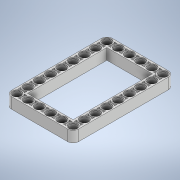
# Autodesk Inventor part: vehicle-adapter
Saved by Autodesk Inventor 2021 (Build 250183000, 183)
## iProperties
Created: 2024-03-15
Part Number: vehicle-adapter
Material: Generic
Document SubType Name: Modeling
Designer: 22hamfri
Density: 1 g/cm^3
Appearance: Default
Author: 22hamfri
Autodesk Inventor part; units mm, degrees
ref_plane "YZ Plane" through (0, 0, 0) normal (1, 0, 0) x (0, 1, 0)
ref_plane "XZ Plane" through (0, 0, 0) normal (0, 1, 0) x (-1, 0, 0)
ref_plane "XY Plane" through (0, 0, 0) normal (0, 0, 1) x (1, 0, 0)
sketch "Sketch1" plane through (0, 0, 0) normal (0, 1, 0) x (-1, 0, 0)
  line L0 (-16.125, 28.08) -> (16.125, 28.08)
  line L1 (16.125, 28.08) -> (16.125, -28.08)
  line L2 (16.125, -28.08) -> (-16.125, -28.08)
  line L3 (-16.125, -28.08) -> (-16.125, 28.08)
  line L4 (-16.125, 28.08) -> (16.125, -28.08) construction
  line L5 (16.125, 28.08) -> (-16.125, -28.08) construction
  circle A0 centre (3.985, -31.88) radius 2.575
  circle A1 centre (3.985, -31.88) radius 3.1
  circle A2 centre (3.985, -31.88) radius 3.8
  circle A3 centre (11.955, -31.88) radius 2.575
  circle A4 centre (11.955, -31.88) radius 3.1
  circle A5 centre (11.955, -31.88) radius 3.8
  circle A6 centre (19.925, -31.88) radius 2.575
  circle A7 centre (19.925, -31.88) radius 3.1
  circle A8 centre (19.925, -31.88) radius 3.8
  circle A9 centre (19.925, -23.91) radius 2.575
  circle A10 centre (19.925, -23.91) radius 3.1
  circle A11 centre (19.925, -23.91) radius 3.8
  circle A12 centre (19.925, -15.94) radius 2.575
  circle A13 centre (19.925, -15.94) radius 3.1
  circle A14 centre (19.925, -15.94) radius 3.8
  circle A15 centre (19.925, -7.97) radius 2.575
  circle A16 centre (19.925, -7.97) radius 3.1
  circle A17 centre (19.925, -7.97) radius 3.8
  circle A18 centre (19.925, 0) radius 2.575
  circle A19 centre (19.925, 0) radius 3.1
  circle A20 centre (19.925, 0) radius 3.8
  line L6 (-23.725, 35.68) -> (23.725, 35.68)
  line L7 (23.725, 35.68) -> (23.725, -35.68)
  line L8 (23.725, -35.68) -> (-23.725, -35.68)
  line L9 (-23.725, -35.68) -> (-23.725, 35.68)
  line L10 (-23.725, 35.68) -> (23.725, -35.68) construction
  line L11 (23.725, 35.68) -> (-23.725, -35.68) construction
  line L12 (23.725, 0) -> (-23.725, 0)
  line L13 (22.225, -3.0249) -> (22.225, -4.9451)
  line L14 (22.225, -10.9949) -> (22.225, -12.9151)
  line L15 (22.225, -18.9649) -> (22.225, -20.8851)
  line L16 (22.225, -26.9349) -> (22.225, -28.8551)
  line L17 (19.925, 0) -> (19.925, -31.88)
  line L18 (17.625, -3.0249) -> (17.625, -4.9451)
  line L19 (17.625, -10.9949) -> (17.625, -12.9151)
  line L20 (17.625, -18.9649) -> (17.625, -20.8851)
  line L21 (17.625, -26.9349) -> (17.625, -28.8551)
  line L22 (16.9001, -34.18) -> (14.9799, -34.18)
  line L23 (8.9301, -34.18) -> (7.0099, -34.18)
  line L24 (19.925, -31.88) -> (3.985, -31.88)
  line L25 (16.9001, -29.58) -> (14.9799, -29.58)
  line L26 (8.9301, -29.58) -> (7.0099, -29.58)
  line L27 (0, 35.68) -> (0, -35.68)
  line L28 (-16.125, 28.08) -> (-16.125, -28.08)
  line L29 (-16.125, -28.08) -> (16.125, -28.08)
  line L30 (16.125, 28.08) -> (-16.125, -28.08) construction
  line L31 (-16.125, 28.08) -> (16.125, -28.08) construction
  circle A21 centre (-3.985, -31.88) radius 2.575
  circle A22 centre (-3.985, -31.88) radius 3.1
  circle A23 centre (-3.985, -31.88) radius 3.8
  circle A24 centre (-11.955, -31.88) radius 2.575
  circle A25 centre (-11.955, -31.88) radius 3.1
  circle A26 centre (-11.955, -31.88) radius 3.8
  circle A27 centre (-19.925, -31.88) radius 2.575
  circle A28 centre (-19.925, -31.88) radius 3.1
  circle A29 centre (-19.925, -31.88) radius 3.8
  circle A30 centre (-19.925, -23.91) radius 2.575
  circle A31 centre (-19.925, -23.91) radius 3.1
  circle A32 centre (-19.925, -23.91) radius 3.8
  circle A33 centre (-19.925, -15.94) radius 2.575
  circle A34 centre (-19.925, -15.94) radius 3.1
  circle A35 centre (-19.925, -15.94) radius 3.8
  circle A36 centre (-19.925, -7.97) radius 2.575
  circle A37 centre (-19.925, -7.97) radius 3.1
  circle A38 centre (-19.925, -7.97) radius 3.8
  circle A39 centre (-19.925, 0) radius 2.575
  circle A40 centre (-19.925, 0) radius 3.1
  circle A41 centre (-19.925, 0) radius 3.8
  line L32 (-23.725, 35.68) -> (-23.725, -35.68)
  line L33 (-23.725, -35.68) -> (23.725, -35.68)
  line L34 (23.725, 35.68) -> (-23.725, -35.68) construction
  line L35 (-23.725, 35.68) -> (23.725, -35.68) construction
  line L36 (-23.725, 0) -> (23.725, 0)
  line L37 (-22.225, -3.0249) -> (-22.225, -4.9451)
  line L38 (-22.225, -10.9949) -> (-22.225, -12.9151)
  line L39 (-22.225, -18.9649) -> (-22.225, -20.8851)
  line L40 (-22.225, -26.9349) -> (-22.225, -28.8551)
  line L41 (-19.925, 0) -> (-19.925, -31.88)
  line L42 (-17.625, -3.0249) -> (-17.625, -4.9451)
  line L43 (-17.625, -10.9949) -> (-17.625, -12.9151)
  line L44 (-17.625, -18.9649) -> (-17.625, -20.8851)
  line L45 (-17.625, -26.9349) -> (-17.625, -28.8551)
  line L46 (-16.9001, -34.18) -> (-14.9799, -34.18)
  line L47 (-8.9301, -34.18) -> (-7.0099, -34.18)
  line L48 (-19.925, -31.88) -> (-3.985, -31.88)
  line L49 (-16.9001, -29.58) -> (-14.9799, -29.58)
  line L50 (-8.9301, -29.58) -> (-7.0099, -29.58)
  line L51 (0.9601, -34.18) -> (-0.9601, -34.18)
  line L52 (0.9601, -29.58) -> (-0.9601, -29.58)
  line L53 (16.125, 28.08) -> (-16.125, 28.08)
  circle A42 centre (3.985, 31.88) radius 2.575
  circle A43 centre (3.985, 31.88) radius 3.1
  circle A44 centre (3.985, 31.88) radius 3.8
  circle A45 centre (11.955, 31.88) radius 2.575
  circle A46 centre (11.955, 31.88) radius 3.1
  circle A47 centre (11.955, 31.88) radius 3.8
  circle A48 centre (19.925, 31.88) radius 2.575
  circle A49 centre (19.925, 31.88) radius 3.1
  circle A50 centre (19.925, 31.88) radius 3.8
  circle A51 centre (19.925, 23.91) radius 2.575
  circle A52 centre (19.925, 23.91) radius 3.1
  circle A53 centre (19.925, 23.91) radius 3.8
  circle A54 centre (19.925, 15.94) radius 2.575
  circle A55 centre (19.925, 15.94) radius 3.1
  circle A56 centre (19.925, 15.94) radius 3.8
  circle A57 centre (19.925, 7.97) radius 2.575
  circle A58 centre (19.925, 7.97) radius 3.1
  circle A59 centre (19.925, 7.97) radius 3.8
  circle A60 centre (19.925, 0) radius 2.575
  circle A61 centre (19.925, 0) radius 3.1
  circle A62 centre (19.925, 0) radius 3.8
  line L54 (23.725, 35.68) -> (-23.725, 35.68)
  line L55 (22.225, 3.0249) -> (22.225, 4.9451)
  line L56 (22.225, 10.9949) -> (22.225, 12.9151)
  line L57 (22.225, 18.9649) -> (22.225, 20.8851)
  line L58 (22.225, 26.9349) -> (22.225, 28.8551)
  line L59 (19.925, 0) -> (19.925, 31.88)
  line L60 (17.625, 3.0249) -> (17.625, 4.9451)
  line L61 (17.625, 10.9949) -> (17.625, 12.9151)
  line L62 (17.625, 18.9649) -> (17.625, 20.8851)
  line L63 (17.625, 26.9349) -> (17.625, 28.8551)
  line L64 (16.9001, 34.18) -> (14.9799, 34.18)
  line L65 (8.9301, 34.18) -> (7.0099, 34.18)
  line L66 (19.925, 31.88) -> (3.985, 31.88)
  line L67 (16.9001, 29.58) -> (14.9799, 29.58)
  line L68 (8.9301, 29.58) -> (7.0099, 29.58)
  circle A63 centre (-3.985, 31.88) radius 2.575
  circle A64 centre (-19.925, 15.94) radius 3.1
  circle A65 centre (-19.925, 31.88) radius 2.575
  circle A66 centre (-19.925, 0) radius 2.575
  circle A67 centre (-19.925, 0) radius 3.1
  circle A68 centre (-19.925, 0) radius 3.8
  circle A69 centre (-19.925, 7.97) radius 2.575
  circle A70 centre (-19.925, 7.97) radius 3.1
  circle A71 centre (-19.925, 7.97) radius 3.8
  circle A72 centre (-19.925, 15.94) radius 2.575
  circle A73 centre (-19.925, 23.91) radius 2.575
  circle A74 centre (-19.925, 23.91) radius 3.1
  circle A75 centre (-19.925, 23.91) radius 3.8
  circle A76 centre (-11.955, 31.88) radius 3.8
  circle A77 centre (-11.955, 31.88) radius 2.575
  circle A78 centre (-11.955, 31.88) radius 3.1
  circle A79 centre (-3.985, 31.88) radius 3.1
  circle A80 centre (-3.985, 31.88) radius 3.8
  circle A81 centre (-19.925, 31.88) radius 3.1
  circle A82 centre (-19.925, 31.88) radius 3.8
  circle A83 centre (-19.925, 15.94) radius 3.8
  line L69 (-16.125, 28.08) -> (16.125, 28.08)
  line L70 (-17.625, 3.0249) -> (-17.625, 4.9451)
  line L71 (-22.225, 3.0249) -> (-22.225, 4.9451)
  line L72 (-17.625, 10.9949) -> (-17.625, 12.9151)
  line L73 (-22.225, 10.9949) -> (-22.225, 12.9151)
  line L74 (-17.625, 18.9649) -> (-17.625, 20.8851)
  line L75 (-19.925, 0) -> (-19.925, 31.88)
  line L76 (-23.725, 35.68) -> (23.725, 35.68)
  line L77 (-22.225, 26.9349) -> (-22.225, 28.8551)
  line L78 (-22.225, 18.9649) -> (-22.225, 20.8851)
  line L79 (-17.625, 26.9349) -> (-17.625, 28.8551)
  line L80 (-16.9001, 29.58) -> (-14.9799, 29.58)
  line L81 (-8.9301, 29.58) -> (-7.0099, 29.58)
  line L82 (-19.925, 31.88) -> (-3.985, 31.88)
  line L83 (-8.9301, 34.18) -> (-7.0099, 34.18)
  line L84 (-16.9001, 34.18) -> (-14.9799, 34.18)
  line L85 (0.9601, 34.18) -> (-0.9601, 34.18)
  line L86 (0.9601, 29.58) -> (-0.9601, 29.58)
  point P0 (0, 0)
  point P1 (19.925, -35.68)
  point P2 (23.725, -31.88)
  point P3 (23.725, 31.88)
  point P4 (19.925, 35.68)
  point P5 (-19.925, 35.68)
  point P6 (-23.725, 31.88)
  point P7 (-23.725, -31.88)
  point P8 (-19.925, -35.68)
  point P9 (-16.825, 0)
  point P10 (-17.35, 0)
  point P11 (-22.5, 0)
  point P12 (-23.025, 0)
  dimension "d0" = 5.15
  dimension "d1" = 6.2
  dimension "d2" = 0.7
  dimension "d5" = 7.97
  dimension "d12" = 7.97
  dimension "d17" = 1.5
  dimension "d18" = 1.5
  dimension "d19" = 7.97
  dimension "d20" = 1.5
  dimension "d21" = 1.5
  constraints: 174 end point, 125 symmetric about line, 80 centre point, 52 point on circle, 9 parallel, 8 midpoint, 6 horizontal, 5 vertical, 4 collinear, 3 tangent, 2 perpendicular, 2 point on line, 95 other
  measures "d0" diameter of A0
  measures "d1" diameter of A1
  measures "d2" radial gap between concentric circles of A1 A2
  measures "d5" distance of L24.end A3.centre
  measures "d12" distance of L17.end A9.centre
  measures "d17" distance between parallel lines of L7 L14
  measures "d18" distance between parallel lines of L8 L22
  measures "d19" distance of L48.end L24.end
  measures "d20" distance between parallel lines of L33 L51
  measures "d21" distance between parallel lines of L2 L52
extrude "Extrusion1" add sketch "Sketch1" against normal mid plane 7.76 contours L3 A75 L79 A82 L80 A76 L0 | A76 L81 A80 L0 | A76 L82 A78 | A75 L75 A74 | L3 A83 L74 A75 | A80 L86 L27 L0 | A80 | A83 L75 A64 | L3 A71 L72 A83 | L27 L86 A44 L0 | A76 L82 A78 | A82 L75 A81 L82 | A71 L75 A70 | L3 A41 L70 A71 | L75 A74 A75 | A44 L68 A47 L0 | A44 | L84 A82 L6 A76 | L82 A81 L75 A82 | A76 L6 A80 L83 | A41 L41 A40 L12 | L12 A40 L75 A41 | L3 A38 L42 A41 | L75 A64 A83 | A75 L9 A82 L77 | L78 A83 L9 A75 | A47 L67 A50 L63 A53 L1 L0 | A47 L66 A46 | L85 A80 L6 L27 | L27 L6 A44 L85 | A20 L18 A17 L1 | L1 A59 L60 A20 | L12 A19 L17 A20 | A20 L59 A19 L12 | L27 L52 A23 L2 | L2 A2 L52 L27 | A38 L41 A37 | L3 A35 L43 A38 | L75 A70 A71 | L73 A71 L9 A83 | L1 A56 L61 A59 | A59 L59 A58 | A17 L19 A14 L1 | A17 L17 A16 | L2 A5 L26 A2 | A2 | A23 L50 A26 L2 | A23 | A35 L41 A34 | L3 A32 L44 A35 | A40 L12 A41 L75 | L41 A41 L12 A40 | L71 A41 L9 A71 | A53 L62 A56 L1 | A53 L59 A52 | A47 L66 A46 | A50 L66 A49 L59 | L6 A47 L65 A44 | A56 L59 A55 | A14 L20 A11 L1 | A14 L17 A13 | A20 L12 A19 L59 | L17 A19 L12 A20 | L2 L1 A11 L21 A8 L25 A5 | A5 L24 A4 | A26 L49 A29 L45 A32 L3 L2 | A26 L48 A25 | L51 A2 L8 L27 | L27 L8 A23 L51 | A32 L41 A31 | L41 A37 A38 | L37 A38 L9 A41 | A47 L6 A50 L64 | A50 L59 A49 L66 | A59 L59 A58 | A11 L17 A10 | A17 L17 A16 | L55 A59 L7 A20 | A20 L7 A17 L13 | L41 A34 A35 | L38 A35 L9 A38 | A53 L59 A52 | A56 L59 A55 | L56 A56 L7 A59 | A14 L17 A13 | A17 L7 A14 L14 | A5 L24 A4 | A8 L17 A7 L24 | L23 A5 L8 A2 | A26 L48 A25 | A29 L48 A28 L41 | A23 L8 A26 L47 | L41 A31 A32 | L39 A32 L9 A35 | L58 A50 L7 A53 | A53 L7 A56 L57 | A11 L17 A10 | A14 L7 A11 L15 | L22 A8 L8 A5 | L24 A7 L17 A8 | A26 L8 A29 L46 | A29 L41 A28 L48 | L40 A29 L9 A32 | A11 L7 A8 L16
extrude "Extrusion2" add sketch "Sketch1" along normal mid plane 6.66 contours A79 | A43 | L82 A77 A78 | A78 L82 A77 | L75 A73 A74 | A74 L75 A73 | L82 A65 L75 A81 | A81 L75 A65 L82 | A40 L41 A39 L12 | L12 A39 L75 A40 | L75 A72 A64 | A64 L75 A72 | L12 A18 L17 A19 | A19 L59 A18 L12 | A1 | A22 | L75 A39 L12 A40 | A40 L12 A39 L41 | L75 A69 A70 | A70 L75 A69 | A19 L12 A18 L59 | L17 A18 L12 A19 | L66 A45 A46 | A46 L66 A45 | L41 A36 A37 | A37 L41 A36 | L66 A48 L59 A49 | A49 L59 A48 L66 | L59 A57 A58 | A58 L59 A57 | L17 A15 A16 | A16 L17 A15 | L41 A33 A34 | A34 L41 A33 | L59 A51 A52 | A52 L59 A51 | L59 A54 A55 | A55 L59 A54 | L17 A12 A13 | A13 L17 A12 | L24 A3 A4 | A4 L24 A3 | L48 A24 A25 | A25 L48 A24 | L41 A30 A31 | A31 L41 A30 | L17 A9 A10 | A10 L17 A9 | L24 A6 L17 A7 | A7 L17 A6 L24 | L48 A27 L41 A28 | A28 L41 A27 L48
extrude "Extrusion3" add sketch "Sketch1" along normal mid plane 4 contours L80 A82 L82 A76 | A76 L82 A80 L81 | A75 L75 A82 L79 | L74 A83 L75 A75 | A80 L85 L27 L86 | L82 A82 L84 A76 | A76 L83 A80 L82 | L72 A71 L75 A83 | A75 L77 A82 L75 | L75 A83 L78 A75 | L27 L85 A44 L86 | L70 A41 L75 A71 | L75 A71 L73 A83 | A44 L66 A47 L68 | L42 A38 L41 A41 | L75 A41 L71 A71 | A47 L66 A50 L67 | A44 L65 A47 L66 | L60 A59 L59 A20 | A20 L17 A17 L18 | L52 A2 L51 L27 | L27 L51 A23 L52 | L43 A35 L41 A38 | L41 A38 L37 A41 | A47 L64 A50 L66 | L61 A56 L59 A59 | A17 L17 A14 L19 | L59 A59 L55 A20 | A20 L13 A17 L17 | L26 A5 L24 A2 | A23 L48 A26 L50 | L44 A32 L41 A35 | L41 A35 L38 A38 | L63 A50 L59 A53 | A53 L59 A56 L62 | L59 A56 L56 A59 | A14 L17 A11 L20 | A17 L14 A14 L17 | L25 A8 L24 A5 | L24 A5 L23 A2 | A26 L48 A29 L49 | A23 L47 A26 L48 | L45 A29 L41 A32 | L41 A32 L39 A35 | L59 A50 L58 A53 | A53 L57 A56 L59 | A11 L17 A8 L21 | A14 L15 A11 L17 | L24 A8 L22 A5 | A26 L46 A29 L48 | L41 A29 L40 A32 | A11 L16 A8 L17
equation "\"d18\" = d17"
equation "\"d19\" = d5"
equation "\"d20\" = d17"
equation "\"d21\" = d17"
body "Solid1"
